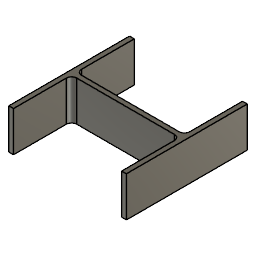
H-294×302×12×12 (Autodesk Fusion 360 design; units mm, degrees)
Autodesk Fusion 360 part; units mm, degrees
sketch "スケッチ1" plane through (0, 0, 0) normal (0, 0, 1) x (1, 0, 0)
  line L0 (294, 151) -> (282, 151)
  line L1 (282, -151) -> (294, -151)
  line L2 (0, 151) -> (0, -151)
  line L3 (12, 19) -> (12, 151)
  line L4 (282, 151) -> (282, 19)
  line L5 (282, -19) -> (282, -151)
  line L6 (12, -151) -> (12, -19)
  line L7 (0, -151) -> (12, -151)
  line L8 (269, 6) -> (25, 6)
  line L9 (25, -6) -> (269, -6)
  line L10 (12, 151) -> (0, 151)
  line L11 (294, -151) -> (294, 151)
  arc A0 (25, -6) -> (12, -19) centre (25, -19) ccw
  arc A1 (12, 19) -> (25, 6) centre (25, 19) ccw
  arc A2 (269, 6) -> (282, 19) centre (269, 19) ccw
  arc A3 (282, -19) -> (269, -6) centre (269, -19) ccw
extrude "押し出し1" add sketch "スケッチ1" along normal blind 100
